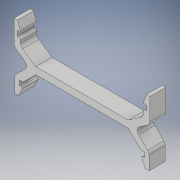
# Autodesk Inventor part: conector-rpi-arduino-improved
Saved by Autodesk Inventor 2019 (Build 230136000, 136)
## iProperties
Created: 2018-06-02
Part Number: conector-rpi-arduino-improved
Material: Generic
Document SubType Name: Modeling
Designer: Alejandro
Density: 1 g/cm^3
Appearance: Default
Author: Alejandro
Autodesk Inventor part; units mm, degrees
ref_plane "YZ Plane" through (0, 0, 0) normal (1, 0, 0) x (0, 1, 0)
ref_plane "XZ Plane" through (0, 0, 0) normal (0, 1, 0) x (-1, 0, 0)
ref_plane "XY Plane" through (0, 0, 0) normal (0, 0, 1) x (1, 0, 0)
sketch "Sketch1" plane through (0, 0, 0) normal (0, 0, 1) x (1, 0, 0)
  line L0 (-28, 11) -> (28, 11)
  line L1 (28, 11) -> (28, 9)
  line L2 (28, 9) -> (-28, 9)
  line L3 (-28, 9) -> (-28, 11)
  line L4 (-27, -7) -> (27, -7)
  line L5 (27, -7) -> (27, -9)
  line L6 (27, -9) -> (-27, -9)
  line L7 (-27, -9) -> (-27, -7)
  line L8 (-20, 1.5) -> (20, 1.5)
  line L9 (20, 1.5) -> (20, -1.5)
  line L10 (20, -1.5) -> (-20, -1.5)
  line L11 (-20, -1.5) -> (-20, 1.5)
  line L12 (26.5, 11) -> (27.8333, 15)
  line L13 (27.8333, 15) -> (29.3333, 15)
  line L14 (29.3333, 15) -> (29.3333, 4.5)
  line L15 (29.3333, 4.5) -> (22.8333, 0)
  line L16 (22.8333, 0) -> (29, -6.1667)
  line L17 (29, -6.1667) -> (29, -13)
  line L18 (29, -13) -> (27.5, -13)
  line L19 (27.5, -13) -> (25.5, -9)
  line L20 (20, -1.5) -> (25.5, -7)
  line L21 (26.5, 9) -> (28, 9)
  line L22 (28, 9) -> (28, 11)
  line L23 (28, 11) -> (26.5, 11)
  line L24 (26.5, 9) -> (26.5, 6)
  line L25 (26.5, 6) -> (20, 1.5)
  point P0 (0, 0)
  point P1 (0, 9)
  point P2 (0, -7)
  point P3 (0, -1.5)
  point P4 (20, 0)
  dimension "d0" = 2
  dimension "d1" = 2
  dimension "d2" = 56
  dimension "d3" = 54
  dimension "d4" = 7
  dimension "d6" = 3
  dimension "d7" = 40
  dimension "d8" = 1.5
  dimension "d9" = 1.5
  dimension "d10" = 1.5
  dimension "d11" = 1.5
  dimension "d13" = 2
  dimension "d14" = 1.5
  dimension "d16" = 4
  dimension "d17" = 4
  dimension "d18" = 1.5
  dimension "d26" = 3
  dimension "d28" = 15
  constraints: 52 end point, 10 parallel, 5 horizontal, 5 perpendicular, 5 point on line, 4 midpoint, 4 vertical alignment, 2 collinear, 2 horizontal alignment, 1 vertical
  measures "d0" distance of L2.end L0.start
  measures "d1" distance of L6.end L4.start
  measures "d2" distance of L0.start L0.end
  measures "d3" distance of L4.start L4.end
  measures "d4" distance from line of point (0, 0) L4
  measures "d6" distance of L8.end L9.end
  measures "d7" distance of L9.end L10.end
  measures "d8" distance of L21.start L1.end
  measures "d9" distance of L0.end L12.start
  measures "d10" distance from line of L5 L19.end
  measures "d11" distance from line of L5 L20.end
  measures "d13" distance between parallel lines of L17 L5
  measures "d14" distance of L12.end L13.end
  measures "d16" distance between parallel lines of L0 L13
  measures "d17" distance between parallel lines of L6 L18
  measures "d18" distance of L17.end L18.end
  measures "d26" distance of L21.start L24.end
  measures "d28" distance from line of point (20, 0) L13
extrude "Extrusion1" add sketch "Sketch1" along normal blind 7 contours L12 L13 L14 L15 L16 L17 L18 L19 L6 L5 L4 L20 L9 L25 L24 L2 L1 L0
mirror "Mirror1" about plane through (0, 0, 0) normal (1, 0, 0) of "Extrusion1"
sketch "Sketch2" plane through (0, 0, 0) normal (0, 0, 1) x (1, 0, 0)
  line L0 (-20, 1.5) -> (-20, -1.5) projected
  line L1 (20, 1.5) -> (20, -1.5) projected
  line L2 (-20, 1.5) -> (20, 1.5)
  line L3 (20, 1.5) -> (20, -1.5)
  line L4 (20, -1.5) -> (-20, -1.5)
  line L5 (-20, -1.5) -> (-20, 1.5)
  point P0 (0, 0)
  constraints: 8 end point, 2 parallel, 1 horizontal, 1 perpendicular
extrude "Extrusion2" add sketch "Sketch2" along normal up to surface (7 mm away)
fillet "Fillet1" radius 2 6 edges at (22.8333, 0, 3.5) (-22.8333, 0, 3.5) (-29.3333, 4.5, 3.5) (29.3333, 4.5, 3.5) (29, -6.1667, 3.5) (-29, -6.1667, 3.5)
fillet "Fillet2" radius 1 4 edges at (-26.5, 9, 3.5) (26.5, 9, 3.5) (25.5, -7, 3.5) (-25.5, -7, 3.5)
fillet "Fillet3" radius 0.5 4 edges at (-26.5, 11, 3.5) (26.5, 11, 3.5) (25.5, -9, 3.5) (-25.5, -9, 3.5)
fillet "Fillet4" radius 2 2 edges at (26.5, 6, 3.5) (-26.5, 6, 3.5)
body "Solid1"
